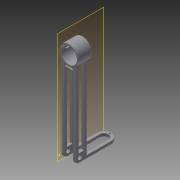
# Autodesk Inventor part: arm
Saved by Autodesk Inventor 2015 (Build 190159000, 159)
## iProperties
Created: 2015-12-15
Part Number: arm
Material: Generic
Document SubType Name: Modeling
Designer: Ross
Density: 1 g/cm^3
Appearance: Default
Author: Ross
Autodesk Inventor part; units mm, degrees
ref_plane "XZ Plane" through (0, 0, 0) normal (0, 1, 0) x (-1, 0, 0)
sketch "Sketch1" plane through (0, 0, 0) normal (0, 0, 1) x (1, 0, 0)
  line L0 (0, 0) -> (15, 0)
  line L1 (0, 0) -> (2.25, 0)
  line L2 (2.25, 0) -> (2.25, 4.6954)
  line L3 (2.25, 0) -> (4.25, 0)
  line L4 (4.25, 0) -> (4.25, 4.6954)
  line L5 (0, 0) -> (4.5, 0)
  line L6 (0, 0) -> (1.7131, 0)
  line L7 (0, 0) -> (2, 0)
  line L8 (2, 0) -> (2, -1.4268)
  line L9 (4.5, 0) -> (4.5, -1.5938)
  line L10 (0, 0) -> (10.5, 0)
  line L11 (10.5, 0) -> (10.5, -1.4268)
  line L12 (0, 0) -> (10.75, 0)
  line L13 (10.75, 0) -> (10.75, 3.2646)
  line L14 (10.75, 0) -> (12.75, 0)
  line L15 (12.75, 0) -> (12.75, 3.2646)
  line L16 (0, 0) -> (13, 0)
  line L17 (13, 0) -> (13, -1.4268)
  line L18 (12.75, 0) -> (12.75, 2)
  line L19 (12.75, 2) -> (10.75, 2)
  line L20 (10.75, 0) -> (12.75, 0)
  line L21 (4.25, 0) -> (4.25, 2)
  line L22 (4.25, 2) -> (2.25, 2)
  dimension "d0" = 15
  dimension "d1" = 2.25
  dimension "d2" = 2
  dimension "d3" = 4.5
  dimension "d4" = 2
  dimension "d5" = 10.5
  dimension "d6" = 10.75
  dimension "d7" = 2
  dimension "d8" = 13
  dimension "d9" = 2
  dimension "d10" = 2
  constraints: 44 end point, 6 perpendicular, 6 point on line, 4 vertical, 1 parallel, 10 other
  measures "d0" distance of L1.start point (15, 0)
  measures "d1" distance of L1.start L1.end
  measures "d2" distance of L1.end L3.end
  measures "d3" distance of L1.start L5.end
  measures "d4" distance of L1.start L7.end
  measures "d5" distance of L1.start L10.end
  measures "d6" distance of L1.start L12.end
  measures "d7" distance of L12.end L14.end
  measures "d8" distance of L1.start L16.end
  measures "d9" distance of L14.end L18.end
  measures "d10" distance of L3.end L21.end
extrude "Extrusion1" add sketch "Sketch1" along normal blind 60
sketch "Sketch2" plane through (2.25, 2, 0) normal (0, 1, 0) x (1, 0, 0)
  line L0 (2, 0) -> (0, 0)
  line L1 (0, 0) -> (0, -6)
  line L2 (0, -6) -> (2, -6)
  line L3 (2, -6) -> (2, 0)
  point P0 (-2.25, 0)
  dimension "d13" = 2
  dimension "d14" = 6
  constraints: 8 end point, 2 parallel, 1 horizontal, 1 perpendicular
  measures "d13" distance of L2.end L1.end
  measures "d14" distance of L1.end L0.end
extrude "Extrusion2" add sketch "Sketch2" along normal blind 4
sketch "Sketch3" plane through (2.25, 0, 60) normal (-1, 0, 0) x (0, 0, 1)
  line L0 (-60, 0) -> (-60, 6)
  line L1 (-60, 0) -> (-60, 6) projected
  line L2 (-60, 6) -> (-54, 6)
  line L3 (-54, 2) -> (-54, 6) projected
  circle A0 centre (-57, 3) radius 1.5
  dimension "d17" = 6
  dimension "d18" = 3
  constraints: 4 end point, 2 point on line, 1 centre point, 1 perpendicular
  measures "d17" distance of L0.start L0.end
  measures "d18" diameter of A0
extrude "Extrusion3" cut sketch "Sketch3" against normal blind 6
sketch "Sketch4" plane through (2.25, 6, 0) normal (0, 1, 0) x (1, 0, 0)
  line L0 (0, 0) -> (2, 0)
  line L1 (2, 0) -> (2, -2)
  line L2 (2, -2) -> (0, -2)
  line L3 (0, -2) -> (0, 0)
  point P0 (-2.25, 0)
  dimension "d22" = 2
  dimension "d23" = 2
  constraints: 8 end point, 2 parallel, 1 horizontal, 1 perpendicular
  measures "d22" distance of L1.end L2.end
  measures "d23" distance of L0.end L1.end
extrude "Extrusion4" add sketch "Sketch4" along normal blind 20
sketch "Sketch5" plane through (10.75, 2, 0) normal (0, 1, 0) x (1, 0, 0)
  line L0 (0, 0) -> (0, -60) projected
  line L1 (2, 0) -> (0, 0)
  line L2 (0, 0) -> (0, -6)
  line L3 (0, -6) -> (2, -6)
  line L4 (2, -6) -> (2, 0)
  point P0 (-10.75, 0)
  dimension "d27" = 6
  constraints: 8 end point, 2 parallel, 1 horizontal, 1 perpendicular, 1 point on line
  measures "d27" distance of L2.end L1.end
extrude "Extrusion5" add sketch "Sketch5" along normal blind 4
sketch "Sketch6" plane through (12.75, 0, 60) normal (1, 0, 0) x (0, 0, -1)
  line L0 (54, 6) -> (60, 0)
  circle A0 centre (57, 3) radius 1.5
  circle A1 centre (57, 3) radius 1.5
  constraints: 2 centre point, 2 end point, 1 coincident, 1 midpoint
extrude "Extrusion6" cut sketch "Sketch6" against normal blind 4
sketch "Sketch7" plane through (10.75, 6, 0) normal (0, 1, 0) x (1, 0, 0)
  line L0 (0, 0) -> (2, 0)
  line L1 (2, 0) -> (2, -2)
  line L2 (2, -2) -> (0, -2)
  line L3 (0, -2) -> (0, 0)
  point P0 (-10.75, 0)
  constraints: 8 end point, 2 parallel, 1 horizontal, 1 perpendicular
extrude "Extrusion7" add sketch "Sketch7" along normal blind 20
ref_plane "Work Plane1" through (0, 0, 0) normal (0, 0, 1) x (1, 0, 0)
sketch "Sketch8" plane through (0, 0, 0) normal (0, 0, 1) x (1, 0, 0)
  arc A0 (12.75, 26) -> (2.25, 26) centre (7.5, 26) ccw
  arc A1 (10.75, 26) -> (4.25, 26) centre (7.5, 26) ccw
  line L0 (12.75, 0) -> (12.75, 26) projected
  line L1 (12.75, 26) -> (10.75, 26)
  line L2 (4.25, 26) -> (2.25, 26)
  line L3 (4.25, 26) -> (2.25, 26)
  line L4 (12.75, 26) -> (10.75, 26)
  line L5 (4.25, 26) -> (2.25, 26)
  arc A2 (10.75, 26) -> (4.25, 26) centre (7.5, 26) ccw
  arc A3 (12.75, 26) -> (2.25, 26) centre (7.5, 26) ccw
  point P0 (0, 0)
  point P1 (12.75, 2)
  constraints: 10 end point, 8 point on circle, 4 centre point, 3 coincident, 2 collinear, 2 horizontal, 1 point on line
extrude "Extrusion8" add sketch "Sketch8" along normal blind 2
ref_plane "Work Plane2" through (0, 0, 60) normal (0, 0, 1) x (1, 0, 0)
sketch "Sketch9" plane through (0, 0, 0) normal (0, 1, 0) x (-1, 0, 0)
  line L0 (-2.25, 60) -> (-12.75, 60)
  line L1 (-7.5, 60) -> (-0.5, 60) construction
  circle A0 centre (-7.5, 67) radius 6
  circle A1 centre (-7.5, 67) radius 7
  point P0 (0, 0)
  constraints: 4 end point, 2 horizontal, 1 centre point, 1 coincident, 1 midpoint, 1 vertical alignment, 2 other
extrude "Extrusion9" add sketch "Sketch9" along normal blind 10
sketch "Sketch10" plane through (0, 0, 60) normal (0, 0, 1) x (1, 0, 0)
  line L0 (2.25, 0) -> (4.25, 0)
  line L1 (4.25, 0) -> (4.25, 2)
  line L2 (4.25, 2) -> (2.25, 2)
  line L3 (2.25, 2) -> (2.25, 0)
  point P0 (0, 0)
  constraints: 8 end point, 2 parallel, 1 horizontal, 1 perpendicular
extrude "Extrusion10" add sketch "Sketch10" along normal blind 1.5
sketch "Sketch11" plane through (0, 0, 61.5) normal (0, 0, 1) x (1, 0, 0)
  line L0 (2.25, 2) -> (3.1699, 2)
  line L1 (3.1699, 2) -> (3.1699, 0)
  line L2 (3.1699, 0) -> (2.25, 0)
  line L3 (2.25, 0) -> (3.1699, 0) projected
  line L4 (2.25, 0) -> (2.25, 2)
  point P0 (0, 0)
  constraints: 8 end point, 2 perpendicular, 1 collinear, 1 horizontal
extrude "Extrusion11" add sketch "Sketch11" along normal blind 1
sketch "Sketch12" plane through (0, 0, 60) normal (0, 0, 1) x (1, 0, 0)
  line L0 (12.75, 0) -> (10.75, 0)
  line L1 (10.75, 0) -> (10.75, 2)
  line L2 (10.75, 2) -> (12.75, 2)
  line L3 (12.75, 2) -> (12.75, 0)
  point P0 (0, 0)
  constraints: 8 end point, 2 parallel, 1 horizontal, 1 perpendicular
extrude "Extrusion12" add sketch "Sketch12" along normal blind 1.5
sketch "Sketch13" plane through (0, 0, 61.5) normal (0, 0, 1) x (1, 0, 0)
  line L0 (12.75, 0) -> (11.8301, 0)
  line L1 (11.8301, 0) -> (11.8301, 2)
  line L2 (11.8301, 2) -> (12.75, 2)
  line L3 (12.75, 2) -> (12.75, 0)
  point P0 (0, 0)
  constraints: 8 end point, 2 parallel, 1 horizontal, 1 perpendicular
extrude "Extrusion13" add sketch "Sketch13" along normal blind 1
sketch "Sketch14" plane through (2.25, 6, 2) normal (0, 0, 1) x (1, 0, 0)
  line L0 (0, 0) -> (2, 0)
  line L1 (2, 0) -> (2, 2)
  line L2 (2, 2) -> (0, 2)
  line L3 (0, 2) -> (0, 0)
  line L4 (8.5, 0) -> (10.5, 0)
  line L5 (10.5, 0) -> (10.5, 2)
  line L6 (10.5, 2) -> (8.5, 2)
  line L7 (8.5, 2) -> (8.5, 0)
  point P0 (-2.25, -6)
  dimension "d52" = 2
  dimension "d53" = 2
  dimension "d54" = 2
  dimension "d55" = 2
  constraints: 16 end point, 4 parallel, 2 horizontal, 2 perpendicular
  measures "d52" distance of L2.end L1.end
  measures "d53" distance of L1.end L0.end
  measures "d54" distance of L6.end L5.end
  measures "d55" distance of L5.end L4.end
extrude "Extrusion14" add sketch "Sketch14" along normal blind 59.5
sketch "Sketch15" plane through (2.25, 6, 61.5) normal (0, 0, 1) x (1, 0, 0)
  line L0 (10.5, 0) -> (9.5801, 0)
  line L1 (9.5801, 0) -> (9.5801, 2)
  line L2 (9.5801, 2) -> (10.5, 2)
  line L3 (10.5, 2) -> (10.5, 0)
  point P0 (-2.25, -6)
  constraints: 8 end point, 2 parallel, 1 horizontal, 1 perpendicular
extrude "Extrusion15" add sketch "Sketch15" along normal blind 1
sketch "Sketch16" plane through (2.25, 6, 61.5) normal (0, 0, 1) x (1, 0, 0)
  line L0 (0, 0) -> (0.9199, 0)
  line L1 (0.9199, 0) -> (0.9199, 2)
  line L2 (0.9199, 2) -> (0, 2)
  line L3 (0, 2) -> (0, 0)
  point P0 (-2.25, -6)
  constraints: 8 end point, 2 parallel, 1 horizontal, 1 perpendicular
extrude "Extrusion16" add sketch "Sketch16" along normal blind 1
fillet "Fillet4" radius 2 2 edges at (3.25, 0, 0) (11.75, 0, 0)
sketch "Sketch17" plane through (0, 0, 0) normal (0, 0, -1) x (-1, 0, 0)
  line L0 (-2.25, 26) -> (-12.75, 26)
  line L1 (-7.5, 26) -> (-7.5, 31.25)
  arc A0 (-2.25, 26) -> (-12.75, 26) centre (-7.5, 26) ccw projected
  circle A1 centre (-7.5, 30.2901) radius 0.5
  point P0 (0, 0)
  dimension "d63" = 1
  constraints: 4 end point, 1 centre point, 1 horizontal, 1 midpoint, 1 point on circle, 1 point on line, 1 vertical
  measures "d63" diameter of A1
extrude "Extrusion17" cut sketch "Sketch17" against normal blind 2 contours A1 L1 | L1 A1
sketch "Sketch18" plane through (10.75, 2, 6) normal (-1, 0, 0) x (0, 0, 1)
  circle A0 centre (52.1755, -1.1123) radius 0.5
  point P0 (-6, -2)
  dimension "d66" = 1
  constraints: 1 centre point
  measures "d66" diameter of A0
extrude "Extrusion18" add sketch "Sketch18" along normal blind 8
ref_plane "Work Plane3" through (0.5, 0, 0) normal (1, 0, 0) x (0, 1, 0)
sketch "Sketch19" plane through (0.5, 0, 0) normal (1, 0, 0) x (0, 1, 0)
  point P0 (0, 0)
sketch "Sketch20" plane through (0.5, 0, 0) normal (1, 0, 0) x (0, 1, 0)
  line L0 (0, 74) -> (0, 62.3699) projected
  line L1 (10, 73) -> (10, 61) projected
  circle A0 centre (5, 67.4828) radius 1.5
  point P0 (0, 0)
  dimension "d70" = 3
  constraints: 1 centre point
  measures "d70" diameter of A0
extrude "Extrusion19" cut sketch "Sketch20" along normal mid plane 10
body "Solid1"
